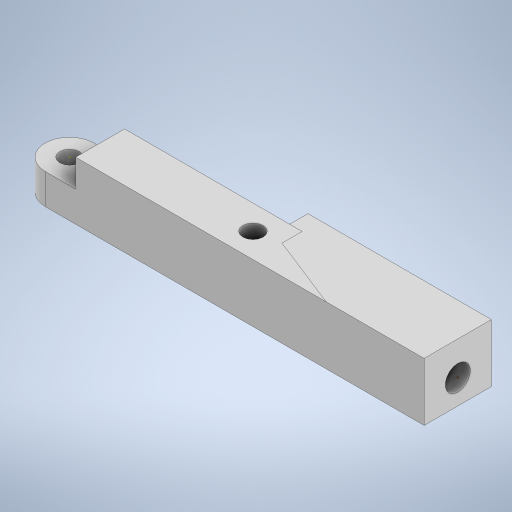
# Autodesk Inventor part: arm
Saved by Autodesk Inventor 2024 (Build 280153000, 153)
## iProperties
Created: 2024-03-04
Part Number: arm
Material: Generic
Document SubType Name: Modeling
Designer: maja6
Density: 1 g/cm^3
Appearance: Default
Author: maja6
Autodesk Inventor part; units mm, degrees
ref_plane "YZ Plane" through (0, 0, 0) normal (1, 0, 0) x (0, 1, 0)
ref_plane "XZ Plane" through (0, 0, 0) normal (0, 1, 0) x (-1, 0, 0)
ref_plane "XY Plane" through (0, 0, 0) normal (0, 0, 1) x (1, 0, 0)
sketch "Sketch1" plane through (0, 0, 0) normal (0, 0, 1) x (1, 0, 0)
  line L0 (0, 0) -> (54, 0)
  circle A0 centre (0, 0) radius 1.55
  line L1 (0, 0) -> (10.0334, 0) construction
  line L2 (0, -2.5) -> (10.0334, -2.5)
  line L3 (10.0334, 2.5) -> (0, 2.5)
  arc A1 (0, 2.5) -> (0, -2.5) centre (0, 0) ccw
  arc A2 (10.0334, -2.5) -> (10.0334, 2.5) centre (10.0334, 0) ccw
  line L4 (0, 0) -> (54, 0) construction
  line L5 (0, -2.5) -> (54, -2.5)
  line L6 (54, 2.5) -> (0, 2.5)
  arc A3 (0, 2.5) -> (0, -2.5) centre (0, 0) ccw
  arc A4 (54, -2.5) -> (54, 2.5) centre (54, 0) ccw
  line L7 (54, 2.5) -> (54, -2.5)
  point P0 (5.0167, 0)
  point P1 (27, 0)
  dimension "d0" = 54
  dimension "d1" = 3.1
  dimension "d2" = 5
  dimension "d3" = 5
  constraints: 20 end point, 8 point on circle, 8 tangent, 5 centre point, 3 equal length, 2 midpoint, 1 coincident, 1 horizontal, 1 point on line, 1 vertical
  measures "d0" distance of L0.start L0.end
  measures "d1" diameter of A0
  measures "d2" diameter of A2
  measures "d3" diameter of A4
extrude "Extrusion1" add sketch "Sketch1" along normal blind 5 contours A2 L6 L7 L0 | L0 L7 L5 A2 | A2 L2 A1 L3
sketch "Sketch2" plane through (0, 0, 5) normal (0, 0, 1) x (1, 0, 0)
  point P0 (0, 0)
sketch "Sketch3" plane through (0, 0, 5) normal (0, 0, 1) x (1, 0, 0)
  circle A0 centre (20.0365, 0) radius 1.5
  point P0 (0, 0)
  dimension "d7" = 3
  constraints: 1 centre point
  measures "d7" diameter of A0
extrude "Extrusion2" cut sketch "Sketch3" against normal blind 5
sketch "Sketch4" plane through (0, 0, 5) normal (0, 0, 1) x (1, 0, 0)
  circle A0 centre (0, 0) radius 1.6
  circle A1 centre (20.0364, 0) radius 1.6
  dimension "d10" = 3.2
  dimension "d11" = 3.2
  constraints: 2 centre point, 1 coincident
  measures "d10" diameter of A0
  measures "d11" diameter of A1
extrude "Extrusion3" cut sketch "Sketch4" against normal blind 5
sketch "Sketch5" plane through (0, 0, 5) normal (0, 0, 1) x (1, 0, 0)
  circle A0 centre (20.0364, 0) radius 1.6 projected
  circle A1 centre (20.0364, 0) radius 1.6
  line L0 (0, 0) -> (24, 0)
  circle A2 centre (24, 0) radius 1.65
  dimension "d14" = 3.2
  dimension "d15" = 24
  dimension "d16" = 3.3
  constraints: 2 centre point, 2 coincident, 2 end point, 1 horizontal
  measures "d14" diameter of A1
  measures "d15" distance of L0.start L0.end
  measures "d16" diameter of A2
extrude "Extrusion4" cut sketch "Sketch5" against normal blind 5 contours A2
extrude "Extrusion5" add sketch "Sketch5" against normal blind 5 contours L0 A0 | A0 L0
sketch "Sketch6" plane through (0, 0, 5) normal (0, 0, 1) x (1, 0, 0)
  line L0 (0, 0) -> (32, 0)
  line L1 (54, 2.5) -> (0, 2.5) projected
  line L2 (0, -2.5) -> (54, -2.5) projected
  line L3 (32, 2.5) -> (54, 2.5)
  line L4 (54, 2.5) -> (54, -2.5)
  line L5 (54, -2.5) -> (32, -2.5)
  line L6 (32, -2.5) -> (32, 2.5)
  dimension "d21" = 32
  constraints: 10 end point, 2 horizontal, 2 parallel, 1 perpendicular, 1 point on line
  measures "d21" distance of L0.start L0.end
extrude "Extrusion6" add sketch "Sketch6" along normal blind 3
sketch "Sketch7" plane through (0, 2.5, 0) normal (0, 1, 0) x (1, 0, 0)
  line L0 (32, -8) -> (54, -8) projected
  line L1 (32, -8) -> (54, -8)
  line L2 (54, -8) -> (54, 0)
  line L3 (54, 0) -> (32, 0)
  line L4 (32, 0) -> (32, -8)
  point P0 (0, 0)
  constraints: 8 end point, 2 parallel, 1 horizontal, 1 perpendicular
extrude "Extrusion7" add sketch "Sketch7" along normal blind 3
sketch "Sketch8" plane through (54, -2.5, 8) normal (1, 0, 0) x (0, 0, -1)
  line L0 (3, 0) -> (0, 0) projected
  line L1 (8, 5) -> (8, 8) projected
  line L2 (0, 0) -> (8, 0)
  line L3 (8, 0) -> (8, 8)
  line L4 (8, 8) -> (0, 8)
  line L5 (0, 8) -> (0, 0)
  point P0 (8, 2.5)
  constraints: 8 end point, 2 parallel, 1 horizontal, 1 perpendicular
extrude "Extrusion8" add sketch "Sketch8" along normal blind 8
sketch "Sketch9" plane through (62, -2.5, 8) normal (1, 0, 0) x (0, 0, -1)
  circle A0 centre (4.0002, 3.9989) radius 2.05
  point P0 (8, 2.5)
  dimension "d28" = 4.1
  constraints: 1 centre point
  measures "d28" diameter of A0
extrude "Extrusion9" cut sketch "Sketch9" against normal blind 25
sketch "Sketch10" plane through (0, 0, 5) normal (0, 0, 1) x (1, 0, 0)
  point P0 (0, 0)
sketch "Sketch11" plane through (0, 0, 5) normal (0, 0, 1) x (1, 0, 0)
  circle A0 centre (0, 0) radius 1.6 projected
  circle A1 centre (0, 0) radius 1.65
  circle A2 centre (24.0003, 0) radius 1.65
  line L0 (0, 0) -> (32.9469, 0) construction
  line L1 (0, -4) -> (32.9469, -4)
  line L2 (32.9469, 4) -> (0, 4)
  arc A3 (0, 4) -> (0, -4) centre (0, 0) ccw
  arc A4 (32.9469, -4) -> (32.9469, 4) centre (32.9469, 0) ccw
  point P0 (16.4734, 0)
  dimension "d31" = 3.3
  dimension "d32" = 3.3
  dimension "d33" = 8
  constraints: 8 end point, 4 centre point, 4 point on circle, 4 tangent, 1 coincident, 1 horizontal, 1 midpoint, 1 parallel
  measures "d31" diameter of A1
  measures "d32" diameter of A2
  measures "d33" diameter of A4
extrude "Extrusion10" add sketch "Sketch11" against normal blind 5 contours A3 L2 A4 L1
sketch "Sketch12" plane through (62, -2.5, 8) normal (1, 0, 0) x (0, 0, -1)
  line L0 (-1.5007, 9.4978) -> (9.5011, 9.4978)
  line L1 (9.5011, 9.4978) -> (9.5011, -1.5)
  line L2 (9.5011, -1.5) -> (-1.5007, -1.5)
  line L3 (-1.5007, -1.5) -> (-1.5007, 9.4978)
  circle A0 centre (4.0002, 3.9989) radius 2.05 projected
  line L4 (-1.5007, 9.4978) -> (9.5011, -1.5) construction
  line L5 (9.5011, 9.4978) -> (-1.5007, -1.5) construction
  circle A1 centre (4.0002, 3.9989) radius 2.05
  point P0 (8, 2.5)
  constraints: 12 end point, 2 midpoint, 2 parallel, 1 centre point, 1 coincident, 1 concentric, 1 horizontal, 1 perpendicular
extrude "Extrusion11" add sketch "Sketch12" against normal blind 30
sketch "Sketch13" plane through (0, -4, 5) normal (0, -1, 0) x (1, 0, 0)
  line L0 (32, -5) -> (32, 0) projected
  line L1 (62, -6.5011) -> (32, -6.5011) projected
  line L2 (32, -5) -> (50, -5)
  line L3 (50, -5) -> (50, -6.5011)
  line L4 (50, -6.5011) -> (32, -6.5011)
  line L5 (32, -6.5011) -> (32, -5)
  point P0 (0, -5)
  dimension "d38" = 18
  constraints: 8 end point, 2 parallel, 1 horizontal, 1 perpendicular, 1 point on line
  measures "d38" distance of L3.end L4.end
extrude "Extrusion12" cut sketch "Sketch13" against normal blind 30
sketch "Sketch14" plane through (62, -4, 9.5007) normal (0, 0, 1) x (1, 0, 0)
  line L0 (-30, 0) -> (-30, 10.9978) projected
  line L1 (0, 0) -> (-30, 0) projected
  line L2 (-30, 5.4989) -> (-16.0053, 0)
  line L3 (-16.0053, 0) -> (-19.5106, -8.9209)
  line L4 (-19.5106, -8.9209) -> (-33.5053, -3.422)
  line L5 (-33.5053, -3.422) -> (-30, 5.4989)
  point P0 (-62, 4)
  constraints: 8 end point, 2 parallel, 1 midpoint, 1 perpendicular, 1 point on line
extrude "Extrusion13" cut sketch "Sketch14" against normal blind 4.5
sketch "Sketch15" plane through (0, 0, 5) normal (0, 0, 1) x (1, 0, 0)
  line L0 (0, 0) -> (30, 0)
  line L1 (32, -4) -> (32, 1.4989) projected
  circle A0 centre (30, 0) radius 1.65
  line L2 (34.0466, 0) -> (31.65, 0)
  line L3 (31.65, 0) -> (31.65, 4.2484)
  line L4 (31.65, 4.2484) -> (34.0466, 4.2484)
  line L5 (34.0466, 4.2484) -> (34.0466, 0)
  dimension "d43" = 30
  dimension "d44" = 3.3
  constraints: 10 end point, 2 parallel, 2 perpendicular, 1 centre point, 1 coincident, 1 horizontal
  measures "d43" distance of L0.start L0.end
  measures "d44" diameter of A0
extrude "Extrusion14" cut sketch "Sketch15" against normal blind 10 contours A0
extrude "Extrusion15" cut sketch "Sketch15" along normal blind 10 contours L3 L4 L5 L2
sketch "Sketch16" plane through (0, 0, 5) normal (0, 0, 1) x (1, 0, 0)
  circle A0 centre (24.0277, 0) radius 2.9708
  point P0 (0, 0)
  constraints: 1 centre point
extrude "Extrusion16" add sketch "Sketch16" against normal blind 5
sketch "Sketch17" plane through (62, -4, -1.5011) normal (0, 0, -1) x (-1, 0, 0)
  line L0 (-2.625, 12.9039) -> (17.8252, 12.9039)
  line L1 (17.8252, 12.9039) -> (17.8252, -5.3634)
  line L2 (17.8252, -5.3634) -> (-2.625, -5.3634)
  line L3 (-2.625, -5.3634) -> (-2.625, 12.9039)
  point P0 (62, 4)
  constraints: 8 end point, 2 parallel, 1 horizontal, 1 perpendicular
extrude "Extrusion17" cut sketch "Sketch17" against normal blind 1.5
sketch "Sketch18" plane through (0, 0, 5) normal (0, 0, 1) x (1, 0, 0)
  circle A0 centre (0, 0) radius 1.6 projected
  line L0 (0, 0) -> (5, 0)
  line L1 (5, 0) -> (47.2457, 0)
  line L2 (47.2457, 0) -> (47.2457, -3.9214)
  line L3 (47.2457, -3.9214) -> (5, -3.9214)
  line L4 (5, -3.9214) -> (5, 0)
  line L5 (32, 4) -> (0, 4) projected
  line L6 (5, 4) -> (47.2457, 4)
  line L7 (47.2457, 4) -> (47.2457, -3.9214)
  line L8 (47.2457, -3.9214) -> (5, -3.9214)
  line L9 (5, -3.9214) -> (5, 4)
  circle A1 centre (30.0062, 0) radius 1.6535
  dimension "d53" = 5
  constraints: 18 end point, 4 parallel, 3 horizontal, 3 point on line, 2 perpendicular, 1 centre point
  measures "d53" distance of L0.start L0.end
extrude "Extrusion18" add sketch "Sketch18" along normal blind 4.5 contours A1 L1 L9 L5 L6 L7 | L1 L2 L3 L4 A1
sketch "Sketch19" plane through (5, -3.9214, 5) normal (0, -1, 0) x (1, 0, 0)
  point P0 (-5, -5)
sketch "Sketch20" plane through (0, 0, 5) normal (0, 0, 1) x (1, 0, 0)
  line L0 (5, -3.9214) -> (5, 4) projected
  line L1 (50, -4) -> (0, -4) projected
  line L2 (5, -2.1351) -> (48.5972, -2.1351)
  line L3 (48.5972, -2.1351) -> (48.5972, -4)
  line L4 (48.5972, -4) -> (5, -4)
  line L5 (5, -4) -> (5, -2.1351)
  point P0 (0, 0)
  constraints: 8 end point, 2 parallel, 2 point on line, 1 horizontal, 1 perpendicular
extrude "Extrusion19" add sketch "Sketch20" along normal blind 4.5
sketch "Sketch21" plane through (62, -4, 9.5007) normal (0, 0, 1) x (1, 0, 0)
  line L0 (-30, 8.2484) -> (-27.9534, 8.2484) projected
  line L1 (-27.9534, 8) -> (-57, 8) projected
  line L2 (-30, 8.2484) -> (-27.9534, 8.2484)
  line L3 (-27.9534, 8.2484) -> (-27.9534, 8)
  line L4 (-27.9534, 8) -> (-30, 8)
  line L5 (-30, 8) -> (-30, 8.2484)
  point P0 (-62, 4)
  constraints: 8 end point, 2 parallel, 1 horizontal, 1 perpendicular
extrude "Extrusion20" add sketch "Sketch21" against normal blind 8
body "Solid1"
